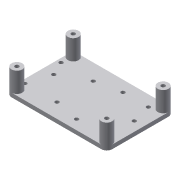
# Autodesk Inventor part: cellSTORM_v5_miniElectronics
Saved by Autodesk Inventor 2019.4 (Build 234330000, 330)
## iProperties
Created: 2020-06-15
Part Number: cellSTORM_v5_miniElectronics
Material: Generic
Document SubType Name: Modeling
Designer: diederichbenedict
Density: 1 g/cm^3
Appearance: White
Author: diederichbenedict
Autodesk Inventor part; units mm, degrees
ref_plane "YZ Plane" through (0, 0, 0) normal (1, 0, 0) x (0, 1, 0)
ref_plane "XZ Plane" through (0, 0, 0) normal (0, 1, 0) x (-1, 0, 0)
ref_plane "XY Plane" through (0, 0, 0) normal (0, 0, 1) x (1, 0, 0)
sketch "Sketch1" plane through (0, 0, 0) normal (0, 1, 0) x (-1, 0, 0)
  line L0 (37.5, 25) -> (-37.5, 25)
  line L1 (-37.5, 25) -> (-37.5, -25)
  line L2 (-37.5, -25) -> (37.5, -25)
  line L3 (37.5, -25) -> (37.5, 25)
  line L4 (37.5, 25) -> (-37.5, -25) construction
  line L5 (-37.5, 25) -> (37.5, -25) construction
  circle A0 centre (29.5, -0.5) radius 2 construction
  circle A1 centre (-30.5, -0.5) radius 2 construction
  circle A2 centre (29.5, -2.5) radius 1.45
  circle A3 centre (-30.5, -2.5) radius 1.45
  point P0 (0, 0)
  dimension "d0" = 75
  dimension "d1" = 50
  dimension "d9" = 2.9
  dimension "d10" = 2.9
  constraints: 12 end point, 2 centre point, 2 midpoint, 2 parallel, 2 vertical alignment, 1 horizontal, 1 perpendicular, 2 other
  measures "d0" distance of L2.end L1.end
  measures "d1" distance of L1.end L0.end
  measures "d9" diameter of A2
  measures "d10" diameter of A3
extrude "Extrusion1" add sketch "Sketch1" along normal blind 3
fillet "Fillet1" radius 4 4 edges at (-37.5, 1.5, 25) (37.5, 1.5, 25) (37.5, 1.5, -25) (-37.5, 1.5, -25)
sketch "Sketch2" plane through (0, 3, 0) normal (0, 1, 0) x (1, 0, 0)
  arc A0 (-33.5, 25) -> (-37.5, 21) centre (-33.5, 21) ccw projected
  line L0 (-37.5, 21) -> (-37.5, -21) projected
  arc A1 (-37.5, -21) -> (-33.5, -25) centre (-33.5, -21) ccw projected
  line L1 (-33.5, -25) -> (33.5, -25) projected
  arc A2 (33.5, -25) -> (37.5, -21) centre (33.5, -21) ccw projected
  line L2 (37.5, -21) -> (37.5, 21) projected
  arc A3 (37.5, 21) -> (33.5, 25) centre (33.5, 21) ccw projected
  line L3 (33.5, 25) -> (-33.5, 25) projected
  circle A4 centre (-33.5, -21) radius 4
  circle A5 centre (-33.5, 21) radius 4
  circle A6 centre (33.5, 21) radius 4
  circle A7 centre (33.5, -21) radius 4
  point P0 (0, 0)
  constraints: 4 centre point, 4 coincident, 4 concentric
extrude "Extrusion2" add sketch "Sketch2" along normal blind 15 contours A5 A0 | A3 A6 | A4 A1 | A2 A7
sketch "Sketch3" plane through (-33.5, 18, -21) normal (0, 1, 0) x (1, 0, 0)
  circle A0 centre (0, 0) radius 4 projected
  circle A1 centre (67, 0) radius 4 projected
  circle A2 centre (67, -42) radius 4 projected
  circle A3 centre (0, -42) radius 4 projected
  point P0 (33.5, -21)
hole "Hole1" at (33.5, 18, -21) at (33.5, 18, 21) at (-33.5, 18, 21) at (-33.5, 18, -21) direction (0, -1, 0) diameter 3 end through all
sketch "Sketch4" plane through (0, 3, 0) normal (0, 1, 0) x (1, 0, 0)
  circle A0 centre (-34.514, 12.9321) radius 1 projected
  circle A1 centre (-10.514, -14.0679) radius 1 projected
  circle A2 centre (-34.514, -14.0679) radius 1 projected
  circle A3 centre (-34.514, 12.9321) radius 1 projected
  circle A4 centre (-10.514, 12.9321) radius 1 projected
  line L0 (-9.014, -15.5679) -> (-9.014, 14.4321) projected
  line L1 (-9.014, 14.4321) -> (-36.014, 14.4321) projected
  line L2 (-36.014, 14.4321) -> (-36.014, -15.5679) projected
  line L3 (-36.014, -15.5679) -> (-9.014, -15.5679) projected
  point P0 (0, 0)
hole "Hole2" at (-10.514, 3, -12.9321) at (-10.514, 3, 14.0679) at (-34.514, 3, 14.0679) at (-34.514, 3, -12.9321) direction (0, -1, 0) diameter 2.9 end through all
sketch "Sketch5" plane through (0, 3, 0) normal (0, 1, 0) x (1, 0, 0)
  circle A0 centre (29.048, -12.3365) radius 0.5 projected
  circle A1 centre (27.048, -12.3365) radius 0.5 projected
  circle A2 centre (25.048, -12.3365) radius 0.5 projected
  circle A3 centre (23.048, -12.3365) radius 0.5 projected
  circle A4 centre (21.048, -12.3365) radius 0.5 projected
  circle A5 centre (19.048, -12.3365) radius 0.5 projected
  circle A6 centre (17.048, -12.3365) radius 0.5 projected
  circle A7 centre (15.048, -12.3365) radius 0.5 projected
  circle A8 centre (13.048, -12.3365) radius 0.5 projected
  circle A9 centre (11.048, -12.3365) radius 0.5 projected
  circle A10 centre (29.048, -14.3365) radius 0.5 projected
  circle A11 centre (27.048, -14.3365) radius 0.5 projected
  circle A12 centre (25.048, -14.3365) radius 0.5 projected
  circle A13 centre (23.048, -14.3365) radius 0.5 projected
  circle A14 centre (21.048, -14.3365) radius 0.5 projected
  circle A15 centre (19.048, -14.3365) radius 0.5 projected
  circle A16 centre (17.048, -14.3365) radius 0.5 projected
  circle A17 centre (15.048, -14.3365) radius 0.5 projected
  circle A18 centre (13.048, -14.3365) radius 0.5 projected
  circle A19 centre (11.048, -14.3365) radius 0.5 projected
  line L0 (36.448, 3.8635) -> (40.048, 3.8635) projected
  line L1 (40.048, 3.8635) -> (40.048, 4.1635) projected
  line L2 (40.048, 4.1635) -> (42.048, 4.1635) projected
  line L3 (42.048, 4.1635) -> (42.048, 15.1635) projected
  line L4 (42.048, 15.1635) -> (5.048, 15.1635) projected
  line L5 (5.048, 15.1635) -> (3.048, 13.1635) projected
  line L6 (3.048, 13.1635) -> (3.048, -14.0365) projected
  line L7 (3.048, -14.0365) -> (5.048, -16.0365) projected
  line L8 (5.048, -16.0365) -> (35.748, -16.0365) projected
  line L9 (35.748, -16.0365) -> (35.748, -13.4365) projected
  line L10 (35.748, -13.4365) -> (36.448, -13.4365) projected
  line L11 (36.448, -13.4365) -> (36.448, -11.3812) projected
  line L12 (36.448, -11.3812) -> (41.4749, -11.3812) projected
  line L13 (41.4749, -11.3812) -> (41.4749, -13.4365) projected
  line L14 (41.4749, -13.4365) -> (42.048, -13.4365) projected
  line L15 (42.048, -13.4365) -> (42.048, -5.1365) projected
  line L16 (42.048, -5.1365) -> (40.048, -5.1365) projected
  line L17 (40.048, -5.1365) -> (40.048, -4.3365) projected
  line L18 (40.048, -4.3365) -> (36.448, -4.3365) projected
  line L19 (36.448, -4.3365) -> (36.448, 3.8635) projected
  line L20 (10.248, -8.4365) -> (10.248, 7.0635) projected
  line L21 (10.248, 7.0635) -> (27.748, 7.0635) projected
  line L22 (27.748, 7.0635) -> (27.748, -8.4365) projected
  line L23 (27.748, -8.4365) -> (10.248, -8.4365) projected
  circle A20 centre (27.048, -17.8067) radius 1.45
  circle A21 centre (7.8064, -17.8067) radius 1.45
  circle A22 centre (7.8064, 16.7636) radius 1.45
  circle A23 centre (26.7811, 16.7636) radius 1.45
  point P0 (0, 0)
  dimension "d25" = 2.9
  dimension "d26" = 2.9
  dimension "d27" = 2.9
  dimension "d28" = 2.9
  constraints: 4 centre point
  measures "d25" diameter of A20
  measures "d26" diameter of A21
  measures "d27" diameter of A22
  measures "d28" diameter of A23
extrude "Extrusion3" cut sketch "Sketch5" against normal blind 15 contours A20 | A21 | A22 | A23
body "Solid1"
